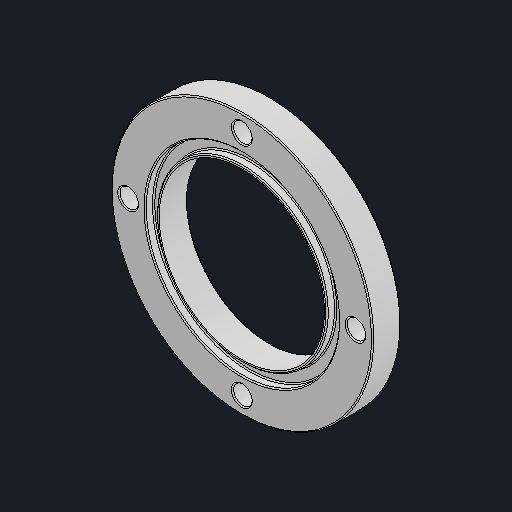
# Autodesk Inventor part: pld_flange_groove_ak
Saved by Autodesk Inventor 2026 (Build 300175050, 175E)
## iProperties
Created: 2025-11-12
Part Number: pld_flange_groove_ak
Material: Generic
Document SubType Name: Modeling
Designer: queezz
Density: 1 g/cm^3
Appearance: Default
Author: queezz
Autodesk Inventor part; units mm, degrees
ref_plane "YZ Plane" through (0, 0, 0) normal (1, 0, 0) x (0, 1, 0)
ref_plane "XZ Plane" through (0, 0, 0) normal (0, 1, 0) x (-1, 0, 0)
ref_plane "XY Plane" through (0, 0, 0) normal (0, 0, 1) x (1, 0, 0)
sketch "Sketch1" plane through (0, 0, 0) normal (0, 0, 1) x (1, 0, 0)
  circle A0 centre (0, 0) radius 46
  circle A1 centre (0, 0) radius 29.05
  dimension "d0" = 58.1
  dimension "d1" = 92
  constraints: 2 centre point, 2 coincident
  measures "d0" diameter of A1
  measures "d1" diameter of A0
extrude "Extrusion1" add sketch "Sketch1" along normal blind 10
sketch "Sketch2" plane through (0, 0, 10) normal (0, 0, 1) x (1, 0, 0)
  circle A0 centre (0, 0) radius 29.05 projected
  circle A1 centre (0, 0) radius 40 construction
  point P0 (0, 40)
  dimension "d4" = 80
  constraints: 1 coincident, 1 vertical alignment, 2 other
hole "Hole1" at (0, 40, 10) direction (0, 0, -1) diameter 6.5 end through all
pattern_circular "Circular Pattern1" count 4 over 360 about axis through (0, 0, 0) along (0, 0, 1) of "Hole1"
sketch "Sketch4" plane through (0, 0, 10) normal (0, 0, 1) x (1, 0, 0)
  circle A0 centre (0, 0) radius 30
  circle A1 centre (0, 0) radius 34
  dimension "d15" = 60
  dimension "d16" = 68
  constraints: 2 centre point, 2 coincident
  measures "d15" diameter of A0
  measures "d16" diameter of A1
extrude "Extrusion2" cut sketch "Sketch4" against normal blind 3
chamfer "Chamfer1" distance 0.4 angle 45 15 edges at (-46, 0, 0) (-46, 0, 10) (0, 43.25, 0) (-43.25, 0, 0) (43.25, 0, 0) (0, -43.25, 0) (43.25, 0, 10) (0, 43.25, 10) (0, -43.25, 10) (-43.25, 0, 10) (-29.05, 0, 0) (-34, 0, 10) (-34, 0, 7) (-30, 0, 7) (-30, 0, 10)
equation "\"d0\" = ID"
equation "\"d1\" = OD"
equation "\"OD\" = 92"
equation "\"ID\" = 58.1"
body "Solid1"
